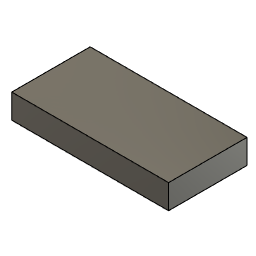
MechanoChip_100um_chip-and-mold (Autodesk Fusion 360 design; units mm, degrees)
Autodesk Fusion 360 part; units mm, degrees
note: some values were not read from the file. Set by a fixed rule: which sketch regions a step uses.
sketch "Sketch1" plane through (0, 0, 0) normal (0, 1, 0) x (1, 0, 0)
  line L0 (-25, 11) -> (25, 11)
  line L1 (25, 11) -> (25, -11)
  line L2 (25, -11) -> (-25, -11)
  line L3 (-25, -11) -> (-25, 11)
  dimension "d56" = 50
  dimension "d57" = 22
  dimension "d59" = 25
  dimension "d126" = 11
  constraint horizontal L0
  constraint vertical L1
  constraint horizontal L2
  constraint vertical L3
  measures "d56" distance of L1.end L2.end
  measures "d57" distance of L0.start L2.end
  measures "d59" distance of origin L3
  measures "d126" distance of origin L0
extrude "Extrude1" add sketch "Sketch1" along normal blind 5 makes body 1
sketch "Sketch4" plane through (-25, 0, 0) normal (-1, 0, 0) x (0, 0, 1)
  line L0 (-11, 0) -> (11, 0)
  line L1 (11, 0) -> (11, 5)
  line L2 (0, 0) -> (0, 11.5) construction
  line L3 (11, 0) -> (-11, 0)
  line L4 (8, 1.5) -> (3.5774, 1.5)
  line L5 (-11, 0) -> (-11, 5)
  line L6 (3, 5) -> (8, 5)
  line L7 (8, 5) -> (8, 1.5)
  arc A0 (2.2783, 3.75) -> (3.5774, 1.5) centre (3.5774, 3) ccw
  line L8 (2.2783, 3.75) -> (3, 5)
  line L9 (-8, 5) -> (-8, 1.5)
  line L10 (-8, 1.5) -> (-3.5774, 1.5)
  line L11 (-3, 5) -> (-8, 5)
  line L12 (-2.2783, 3.75) -> (-3, 5)
  arc A1 (-3.5774, 1.5) -> (-2.2783, 3.75) centre (-3.5774, 3) ccw
  point P0 (1.9896, 3.25)
  point P1 (9.0104, 3.25)
  dimension "d145" = 1.5
  dimension "d217" = 5
  dimension "d218" = 8
  dimension "d277" = 3.5
  dimension "d284" = 1.75
  dimension "d290" = 3
  dimension "d296" = 120
  dimension "d297" = 2
  constraint coincident L2.start origin
  constraint coincident L4.end A0.end
  constraint tangent A0 L8
  constraint tangent L4 A0
  constraint symmetric L2 L4.end L10.end
  constraint symmetric L2 L4.start L9.end
  constraint symmetric L2 L6.start L11.start
  constraint symmetric L2 L6.end L9.start
  constraint symmetric L2 A0.start L12.start
  constraint symmetric L2 A0 A1
  measures "d145" distance of L3 L4
  measures "d217" distance of L6.start L6.end
  measures "d218" distance of L2 L6.end
  measures "d277" distance of L4 L6
  measures "d284" distance of L4 P1
  measures "d290" distance of L1 L4.start
  measures "d296" angle of L6 L8
  measures "d297" vertical distance of L6.start A0.centre
extrude "Extrusion13" cut sketch "Sketch4" against normal blind 10.25 from surface at -27.5 bodies 1
extrude "Extrusion11" cut sketch "Sketch4" against normal blind 10.25 from surface at -12.25 bodies 1
sketch "Sketch7" plane through (0, 5, 0) normal (0, 1, 0) x (-1, 0, 0)
  line L0 (12.5, 5.5) -> (15, 5.5)
  line L1 (15, 5.5) -> (19.125, 0)
  line L2 (12.5, 6.5) -> (15.5, 6.5)
  line L3 (15.5, 6.5) -> (20, 0.5)
  line L4 (20, 0.5) -> (22, 0.5)
  line L5 (0, 0) -> (17.0355, 0) construction
  line L6 (12.5, -6.5) -> (15.5, -6.5)
  line L7 (12.5, -5.5) -> (15, -5.5)
  line L8 (15, -5.5) -> (19.125, 0)
  line L9 (15.5, -6.5) -> (20, -0.5)
  line L10 (20, -0.5) -> (22, -0.5)
  arc A0 (22, -0.5) -> (22, 0.5) centre (22, 0) ccw
  line L11 (12.5, -6.5) -> (12.5, -5.5)
  line L12 (12.5, 5.5) -> (12.5, 6.5)
  line L13 (0, -9.0761) -> (0, 9.0761)
  line L14 (-15, -5.5) -> (-19.125, 0)
  line L15 (-12.5, -6.5) -> (-12.5, -5.5)
  arc A1 (-22, 0.5) -> (-22, -0.5) centre (-22, 0) ccw
  line L16 (-20, -0.5) -> (-22, -0.5)
  line L17 (-12.5, 6.5) -> (-15.5, 6.5)
  line L18 (-15, 5.5) -> (-19.125, 0)
  line L19 (-12.5, 5.5) -> (-15, 5.5)
  line L20 (-12.5, -6.5) -> (-15.5, -6.5)
  line L21 (-15.5, 6.5) -> (-20, 0.5)
  line L22 (-20, 0.5) -> (-22, 0.5)
  line L23 (-12.5, -5.5) -> (-15, -5.5)
  line L24 (-15.5, -6.5) -> (-20, -0.5)
  line L25 (-12.5, 5.5) -> (-12.5, 6.5)
  line L26 (12.75, 8) -> (12.75, 3)
  line L27 (2.5, 3) -> (2.5, 8)
  line L28 (-2.5, 8) -> (-2.5, 3)
  line L29 (-12.75, 3) -> (-12.75, 8)
  line L30 (25, 11) -> (-25, 11)
  line L31 (-25, 11) -> (-25, -11)
  line L32 (-25, -11) -> (25, -11)
  line L33 (25, -11) -> (25, 11)
  line L34 (25, 11) -> (25, -11)
  line L35 (12.75, 3) -> (2.5, 3)
  line L36 (2.5, 8) -> (12.75, 8)
  line L37 (-2.5, 3) -> (-12.75, 3)
  line L38 (-12.75, 8) -> (-2.5, 8)
  line L39 (-2.5, -8) -> (-12.75, -8)
  line L40 (-12.75, -8) -> (-12.75, -3)
  line L41 (-12.75, -3) -> (-2.5, -3)
  line L42 (-2.5, -3) -> (-2.5, -8)
  line L43 (12.75, -8) -> (2.5, -8)
  line L44 (2.5, -8) -> (2.5, -3)
  line L45 (2.5, -3) -> (12.75, -3)
  line L46 (12.75, -3) -> (12.75, -8)
  dimension "d47" = 5.5
  dimension "d48" = 1
  dimension "d49" = 1
  dimension "d50" = 0.5
  dimension "d51" = 1
  dimension "d55" = 2
  dimension "d61" = 3
  dimension "d125" = 12.5
  dimension "d238" = 106.3
  dimension "d256" = 3
  dimension "d257" = 5.5
  constraint horizontal L0
  constraint horizontal L2
  constraint parallel L2 L4
  constraint horizontal L5
  constraint coincident L1.end L5
  constraint parallel L1 L3
  constraint symmetric L0.start L5 L7.start
  constraint symmetric L0.end L5 L7.end
  constraint symmetric L1.end L5 L8.end
  constraint symmetric L2.start L5 L6.start
  constraint symmetric L2.end L5 L6.end
  constraint symmetric L3.end L5 L9.end
  constraint symmetric L4.end L5 L10.end
  constraint coincident L4 A0.end
  constraint coincident L10 A0.start
  constraint coincident L10.end A0.start
  constraint vertical L11
  constraint perpendicular L5 L13
  constraint symmetric L0.start L13 L19.start
  constraint symmetric L0.end L13 L18.start
  constraint symmetric L1.end L13 L14.end
  constraint symmetric L2.start L13 L17.start
  constraint symmetric L2.end L13 L17.end
  constraint symmetric L3.end L13 L21.end
  constraint symmetric L4.end L13 A1.start
  constraint symmetric L6.start L13 L15.start
  constraint symmetric L6.end L13 L20.end
  constraint symmetric L7.start L13 L15.end
  constraint symmetric L7.end L13 L14.start
  constraint symmetric L9.end L13 L16.start
  constraint symmetric L10.end L13 A1.end
  constraint symmetric A0 L13 A1
  constraint midpoint L13 L5.start
  constraint coincident origin L5
  measures "d47" distance of L0 L5
  measures "d48" distance of L0 L2
  measures "d49" distance of L1 L3
  measures "d50" distance of L4 L5
  measures "d51" diameter of A0
  measures "d55" distance of L9.end L10.end
  measures "d61" distance of L2.start L2.end
  measures "d125" distance of L5.start L12
  measures "d256" distance of A0.centre L34
  measures "d257" distance of L5.start L7
extrude "Extrusion9" cut sketch "Sketch7" against normal blind 1 contours L14 A1 L16 L17 L18 L19 L20 L21 L22 L23 L24 L29 L40 | L15 L20 L23 L40 | L17 L19 L25 L29 bodies 1
extrude "Extrude6" cut sketch "Sketch7" against normal blind 1 contours L0 L2 L12 L26 | L0 L1 L2 L3 L4 L6 L7 L8 L9 L10 A0 L26 L46 | L6 L7 L11 L46 bodies 1
sketch "Sketch6" plane through (0, 5, 0) normal (0, 1, 0) x (-1, 0, 0)
  line L0 (-37.5, 12.5) -> (37.5, 12.5)
  line L1 (37.5, 12.5) -> (37.5, -12.5)
  line L2 (37.5, -12.5) -> (-37.5, -12.5)
  line L3 (-37.5, -12.5) -> (-37.5, 12.5)
  line L4 (15.5, -6.5) -> (12.75, -6.5)
  line L5 (12.75, -5.5) -> (15, -5.5)
  line L6 (15, -5.5) -> (19.125, 0)
  line L7 (19.125, 0) -> (15, 5.5)
  line L8 (15, 5.5) -> (12.75, 5.5)
  line L9 (12.75, -6.5) -> (12.75, -8)
  line L10 (12.75, 6.5) -> (15.5, 6.5)
  line L11 (15.5, 6.5) -> (20, 0.5)
  line L12 (20, 0.5) -> (22, 0.5)
  arc A0 (22, -0.5) -> (22, 0.5) centre (22, 0) ccw
  line L13 (22, -0.5) -> (20, -0.5)
  line L14 (20, -0.5) -> (15.5, -6.5)
  line L15 (25, 11) -> (-25, 11)
  line L16 (-25, 11) -> (-25, -11)
  line L17 (-25, -11) -> (25, -11)
  line L18 (25, -11) -> (25, 11)
  line L19 (-12.75, -6.5) -> (-15.5, -6.5)
  line L20 (-15.5, -6.5) -> (-20, -0.5)
  line L21 (-20, -0.5) -> (-22, -0.5)
  arc A1 (-22, 0.5) -> (-22, -0.5) centre (-22, 0) ccw
  line L22 (-22, 0.5) -> (-20, 0.5)
  line L23 (-20, 0.5) -> (-15.5, 6.5)
  line L24 (-15.5, 6.5) -> (-12.75, 6.5)
  line L25 (-2.5, 8) -> (-2.5, 3)
  line L26 (-12.75, 6.5) -> (-12.75, 8)
  line L27 (-12.75, 5.5) -> (-15, 5.5)
  line L28 (-15, 5.5) -> (-19.125, 0)
  line L29 (-19.125, 0) -> (-15, -5.5)
  line L30 (-15, -5.5) -> (-12.75, -5.5)
  line L31 (12.75, 3) -> (2.5, 3)
  line L32 (2.5, -8) -> (2.5, -3)
  line L33 (2.5, 8) -> (12.75, 8)
  line L34 (12.75, 8) -> (12.75, 6.5)
  line L35 (-12.75, 8) -> (-2.5, 8)
  line L36 (-2.5, 3) -> (-12.75, 3)
  line L37 (-12.75, 3) -> (-12.75, 5.5)
  line L38 (-12.75, -5.5) -> (-12.75, -3)
  line L39 (-12.75, -3) -> (-2.5, -3)
  line L40 (-2.5, -3) -> (-2.5, -8)
  line L41 (-2.5, -8) -> (-12.75, -8)
  line L42 (-12.75, -8) -> (-12.75, -6.5)
  line L43 (12.75, -8) -> (2.5, -8)
  line L44 (2.5, -3) -> (12.75, -3)
  line L45 (12.75, -3) -> (12.75, -5.5)
  line L46 (12.75, 5.5) -> (12.75, 3)
  line L47 (2.5, 3) -> (2.5, 8)
  dimension "d252" = 75
  dimension "d253" = 25
  dimension "d254" = 12.5
  dimension "d255" = 37.5
  constraint horizontal L0
  constraint vertical L1
  constraint horizontal L2
  constraint vertical L3
  measures "d252" distance of L0.start L0.end
  measures "d253" distance of L0.start L2.end
  measures "d254" distance of origin L0
  measures "d255" distance of origin L3
extrude "Extrude5" add sketch "Sketch6" along normal blind 1 separate body contours L0 L1 L2 L3 | L4 L5 L6 L7 L8 L9 L10 L11 L12 A0 L13 L14 L31 L32 L33 L34 L43 L44 L45 L46 L47 | L15 L16 L17 L18 | L19 L20 L21 A1 L22 L23 L24 L25 L26 L27 L28 L29 L30 L35 L36 L37 L38 L39 L40 L41 L42 makes body 2
sketch "Sketch20" plane through (0, 5, 0) normal (0, 1, 0) x (-1, 0, 0)
  circle A0 centre (-7.625, 0) radius 1.25
  line L0 (0, -4) -> (0, 4) construction
  circle A1 centre (7.625, 0) radius 1.25
  line L1 (-1.5, -3.5) -> (-1.5, -8)
  line L2 (-20, -0.5) -> (-22, -0.5)
  line L3 (15.5, -6.5) -> (12.75, -6.5)
  line L4 (12.75, -5.5) -> (15, -5.5)
  line L5 (15, -5.5) -> (19.125, 0)
  line L6 (19.125, 0) -> (15, 5.5)
  line L7 (15, 5.5) -> (12.75, 5.5)
  line L8 (12.75, -6.5) -> (12.75, -8)
  line L9 (12.75, 6.5) -> (15.5, 6.5)
  line L10 (15.5, 6.5) -> (20, 0.5)
  line L11 (20, 0.5) -> (22, 0.5)
  arc A2 (22, -0.5) -> (22, 0.5) centre (22, 0) ccw
  line L12 (22, -0.5) -> (20, -0.5)
  line L13 (20, -0.5) -> (15.5, -6.5)
  line L14 (25, 11) -> (-25, 11)
  line L15 (-25, 11) -> (-25, -11)
  line L16 (-25, -11) -> (25, -11)
  line L17 (25, -11) -> (25, 11)
  line L18 (-12.75, -6.5) -> (-15.5, -6.5)
  line L19 (-15.5, -6.5) -> (-20, -0.5)
  line L20 (-20, -0.5) -> (-22, -0.5)
  arc A3 (-22, 0.5) -> (-22, -0.5) centre (-22, 0) ccw
  line L21 (-22, 0.5) -> (-20, 0.5)
  line L22 (-20, 0.5) -> (-15.5, 6.5)
  line L23 (-15.5, 6.5) -> (-12.75, 6.5)
  line L24 (-2.5, 8) -> (-2.5, 3)
  line L25 (-12.75, 6.5) -> (-12.75, 8)
  line L26 (-12.75, 5.5) -> (-15, 5.5)
  line L27 (-15, 5.5) -> (-19.125, 0)
  line L28 (-19.125, 0) -> (-15, -5.5)
  line L29 (-15, -5.5) -> (-12.75, -5.5)
  line L30 (12.75, 3) -> (2.5, 3)
  line L31 (2.5, -8) -> (2.5, -3)
  line L32 (2.5, 8) -> (12.75, 8)
  line L33 (12.75, 8) -> (12.75, 6.5)
  line L34 (-12.75, 8) -> (-2.5, 8)
  line L35 (-2.5, 3) -> (-12.75, 3)
  line L36 (-12.75, 3) -> (-12.75, 5.5)
  line L37 (-12.75, -5.5) -> (-12.75, -3)
  line L38 (-12.75, -3) -> (-2.5, -3)
  line L39 (-2.5, -3) -> (-2.5, -8)
  line L40 (-2.5, -8) -> (-12.75, -8)
  line L41 (-12.75, -8) -> (-12.75, -6.5)
  line L42 (12.75, -8) -> (2.5, -8)
  line L43 (2.5, -3) -> (12.75, -3)
  line L44 (12.75, -3) -> (12.75, -5.5)
  line L45 (12.75, 5.5) -> (12.75, 3)
  line L46 (2.5, 3) -> (2.5, 8)
  dimension "d259" = 2.5
  dimension "d271" = 6.125
  dimension "d272" = 0.5
  constraint vertical L0
  constraint symmetric A0 L0 A1
  constraint coincident origin L0
  measures "d259" diameter of A0
  measures "d271" distance of A0.centre L1
  measures "d272" distance of A0.centre L2
sketch "Sketch21" plane through (0, 5, 0) normal (0, 1, 0) x (-1, 0, 0)
  line L0 (-15.625, 0.25) -> (-8.8497, 0.25)
  circle A0 centre (-7.625, 0) radius 1.25
  line L1 (-15.625, -0.25) -> (-8.8497, -0.25)
  line L2 (-7.625, 2.137) -> (-7.625, -2.2419) construction
  arc A1 (-15.625, 0.25) -> (-15.625, -0.25) centre (-15.625, 0) ccw
  line L3 (0, 3.3559) -> (0, -2.8559) construction
  arc A2 (15.625, -0.25) -> (15.625, 0.25) centre (15.625, 0) ccw
  line L4 (-6.4003, -0.25) -> (0, -0.25)
  line L5 (0, 0.25) -> (-6.4003, 0.25)
  line L6 (0, -0.25) -> (0, 0.25)
  line L7 (6.4003, -0.25) -> (0, -0.25)
  line L8 (0, 0.25) -> (6.4003, 0.25)
  line L9 (0, -0.25) -> (0, 0.25)
  line L10 (15.625, -0.25) -> (8.8497, -0.25)
  line L11 (15.625, 0.25) -> (8.8497, 0.25)
  arc A3 (15.625, -0.25) -> (15.625, 0.25) centre (15.625, 0) ccw
  circle A4 centre (7.625, 0) radius 1.25
  line L12 (15.5, -6.5) -> (12.75, -6.5)
  line L13 (12.75, -5.5) -> (15, -5.5)
  line L14 (15, -5.5) -> (19.125, 0)
  line L15 (19.125, 0) -> (15, 5.5)
  line L16 (15, 5.5) -> (12.75, 5.5)
  line L17 (12.75, -6.5) -> (12.75, -8)
  line L18 (12.75, 6.5) -> (15.5, 6.5)
  line L19 (15.5, 6.5) -> (20, 0.5)
  line L20 (20, 0.5) -> (22, 0.5)
  arc A5 (22, -0.5) -> (22, 0.5) centre (22, 0) ccw
  line L21 (22, -0.5) -> (20, -0.5)
  line L22 (20, -0.5) -> (15.5, -6.5)
  line L23 (25, 11) -> (-25, 11)
  line L24 (-25, 11) -> (-25, -11)
  line L25 (-25, -11) -> (25, -11)
  line L26 (25, -11) -> (25, 11)
  line L27 (-12.75, -6.5) -> (-15.5, -6.5)
  line L28 (-15.5, -6.5) -> (-20, -0.5)
  line L29 (-20, -0.5) -> (-22, -0.5)
  arc A6 (-22, 0.5) -> (-22, -0.5) centre (-22, 0) ccw
  line L30 (-22, 0.5) -> (-20, 0.5)
  line L31 (-20, 0.5) -> (-15.5, 6.5)
  line L32 (-15.5, 6.5) -> (-12.75, 6.5)
  line L33 (-2.5, 8) -> (-2.5, 3)
  line L34 (-12.75, 6.5) -> (-12.75, 8)
  line L35 (-12.75, 5.5) -> (-15, 5.5)
  line L36 (-15, 5.5) -> (-19.125, 0)
  line L37 (-19.125, 0) -> (-15, -5.5)
  line L38 (-15, -5.5) -> (-12.75, -5.5)
  line L39 (12.75, 3) -> (2.5, 3)
  line L40 (2.5, -8) -> (2.5, -3)
  line L41 (2.5, 8) -> (12.75, 8)
  line L42 (12.75, 8) -> (12.75, 6.5)
  line L43 (-12.75, 8) -> (-2.5, 8)
  line L44 (-2.5, 3) -> (-12.75, 3)
  line L45 (-12.75, 3) -> (-12.75, 5.5)
  line L46 (-12.75, -5.5) -> (-12.75, -3)
  line L47 (-12.75, -3) -> (-2.5, -3)
  line L48 (-2.5, -3) -> (-2.5, -8)
  line L49 (-2.5, -8) -> (-12.75, -8)
  line L50 (-12.75, -8) -> (-12.75, -6.5)
  line L51 (12.75, -8) -> (2.5, -8)
  line L52 (2.5, -3) -> (12.75, -3)
  line L53 (12.75, -3) -> (12.75, -5.5)
  line L54 (12.75, 5.5) -> (12.75, 3)
  line L55 (2.5, 3) -> (2.5, 8)
  point P0 (-7.625, 0)
  dimension "d260" = 0.5
  dimension "d261" = 0.25
  dimension "d262" = 8
  dimension "d267" = 0.5
  dimension "d268" = 0.25
  constraint tangent L0 A1
  constraint horizontal L0
  constraint coincident L0.end A0
  constraint coincident A0 L1.end
  constraint parallel L0 L1
  constraint tangent L1 A1
  constraint vertical L2
  constraint coincident L2 P0
  constraint vertical L3
  constraint symmetric L0.start L3 A2.end
  constraint symmetric L1.start L3 A2.start
  constraint symmetric A1 L3 A2
  constraint coincident L3 origin
  constraint coincident A0 L4.start
  constraint coincident L3 L4.end
  constraint perpendicular L3 L4
  constraint midpoint L3 L5.start
  constraint coincident A0 L5.end
  constraint parallel L4 L5
  constraint symmetric L0.end L3 L11.end
  constraint symmetric L1.end L3 L10.end
  constraint symmetric A1 L3 A3
  constraint symmetric L3 L4.start L7.start
  constraint symmetric L3 L4.end L6.start
  constraint symmetric L3 L5.start L6.end
  constraint symmetric L3 L5.end L8.end
  constraint symmetric A0 L3 A4
  measures "d260" diameter of A1
  measures "d261" distance of L0 P0
  measures "d262" distance of A1.centre P0
  measures "d267" distance of L4 L5
  measures "d268" distance of origin L4
extrude "Extrude15" cut sketch "Sketch20" sketch "Sketch21" against normal blind 0.1 contours A1 of sketch 2 contours A0 bodies 1
extrude "Extrude16" cut sketch "Sketch21" against normal blind 0.5 contours L0 A0 L1 A1 | A0 L4 L5 L6 L9 | L6 L7 L8 L9 A4 | A2 L10 L11 A3 A4 bodies 1
fillet "Fillet1" radius 1 4 edges at (8.875, 4.5, 0) (6.375, 4.5, 0) (-6.375, 4.5, 0) (-8.875, 4.5, 0) on bodies 1
sketch "Sketch22" plane through (0, 0, 0) normal (0, -1, 0) x (-1, 0, 0)
  line L0 (29, -14.5) -> (-29, -14.5)
  line L1 (-29, -14.5) -> (-29, 14.5)
  line L2 (-29, 14.5) -> (29, 14.5)
  line L3 (29, 14.5) -> (29, -14.5)
  dimension "d299" = 29
  dimension "d300" = 58
  dimension "d301" = 29
  dimension "d302" = 14.5
  constraint parallel L0 L2
  constraint parallel L1 L3
  constraint perpendicular L1 L2
  constraint horizontal L0
  measures "d299" distance of L0.end L1.end
  measures "d300" distance of L0.start L0.end
  measures "d301" distance of origin L1
  measures "d302" distance of origin L0
extrude "Extrude17" add sketch "Sketch22" against normal blind 9 separate body makes body 3
combine "Combine1" operation cut target body 3 tool bodies 1 keep tools result as body 4 in component "printable_mold"
sketch "Sketch23" plane through (-29, 0, 0) normal (-1, 0, 0) x (0, 0, 1)
  line L0 (-14.5, 0) -> (14.5, 0)
  line L1 (14.5, 0) -> (14.5, 9)
  line L2 (14.5, 9) -> (-14.5, 9)
  line L3 (-14.5, 9) -> (-14.5, 0)
  line L4 (10.9863, 3.06) -> (11.9863, 3.06)
  line L5 (11.9863, 3.06) -> (11.9863, 7.06)
  line L6 (11.9863, 7.06) -> (10.9863, 7.06)
  line L7 (10.9863, 7.06) -> (10.9863, 3.06)
  circle A0 centre (7.9847, 5.0026) radius 1.5
  circle A1 centre (7.9847, 5.0026) radius 2
  circle A2 centre (2.9847, 5.0026) radius 2
  circle A3 centre (2.9847, 5.0026) radius 1.5
  line L8 (-5, 0) -> (-9, 0)
  line L9 (-9, 0) -> (-9, 5)
  line L10 (-9, 5) -> (-5, 5)
  line L11 (-5, 5) -> (-5, 0)
  dimension "d306" = 1
  dimension "d307" = 4
  dimension "d308" = 0.5
  dimension "d309" = 3
  dimension "d310" = 0.5
  dimension "d311" = 3
  dimension "d316" = 5
  constraint horizontal L4
  constraint vertical L5
  constraint horizontal L6
  constraint vertical L7
  constraint horizontal L8
  constraint vertical L9
  constraint horizontal L10
  constraint vertical L11
  constraint coincident L0 L8.start
  measures "d306" distance of L4.start L4.end
  measures "d307" distance of L4.start L6.end
  measures "d309" diameter of A0
  measures "d311" diameter of A3
  measures "d316" distance of L8.start L10.end
extrude "Extrude1'" add sketch "Sketch23" along normal blind 1 contours L4 L5 L6 L7 | A1 | A2 bodies 4 in component "printable_mold"
extrude "Extrusion2" cut sketch "Sketch23" against normal blind 4 contours L0 L8 L9 L10 L11 bodies 4 in component "printable_mold"
component "printable_mold" placed x (1, 0, 0) y (0, 1, 0) z (0, 0, 1) at (0, 0, 0)
hidden bodies 1 2 3
equation "d254 = d253 / 2"
equation "d255 = d252 / 2"
equation "d284 = d277 / 2"
equation "d301 = d300 / 2"
equation "d302 = d299 / 2"
named bodies: "PDMS_block", "glass slide", "mold_base_shape"
